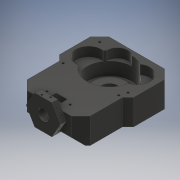
# Autodesk Inventor part: AC01
Saved by Autodesk Inventor 2017 (Build 210142000, 142)
## iProperties
Created: 2019-08-28
Part Number: AC01
Material: ABS Plastic
Document SubType Name: Modeling
Designer: Dell
Density: 1.06 g/cm^3
Appearance: Smooth - Black
Mass: 650.068 g
Surface Area: 1285.03 cm^2
Volume: 613.271 cm^3
Author: Dell
Autodesk Inventor part; units mm, degrees
ref_plane "YZ Plane" through (0, 0, 0) normal (1, 0, 0) x (0, 1, 0)
ref_plane "XZ Plane" through (0, 0, 0) normal (0, 1, 0) x (-1, 0, 0)
ref_plane "XY Plane" through (0, 0, 0) normal (0, 0, 1) x (1, 0, 0)
sketch "Sketch1" plane through (0, 0, 0) normal (0, 0, 1) x (1, 0, 0)
  circle A0 centre (0, 0) radius 17.5
  circle A1 centre (0, 0) radius 82.5
  circle A2 centre (41.5, 0) radius 2
  circle A3 centre (29.3449, 29.3449) radius 2
  circle A4 centre (0, 41.5) radius 2
  circle A5 centre (-29.3449, 29.3449) radius 2
  circle A6 centre (-41.5, 0) radius 2
  circle A7 centre (-29.3449, -29.3449) radius 2
  circle A8 centre (0, -41.5) radius 2
  circle A9 centre (29.3449, -29.3449) radius 2
  dimension "d0" = 35
  dimension "d1" = 165
  dimension "d2" = 4
  dimension "d3" = 41.5
  dimension "d6" = 360
  constraints: 10 centre point, 2 coincident, 1 horizontal alignment, 17 other
  measures "d0" diameter of A0
  measures "d1" diameter of A1
  measures "d2" diameter of A2
  measures "d3" distance of A2.centre point (0, 0)
extrude "Extrusion1" add sketch "Sketch1" along normal blind 15
sketch "Sketch5" plane through (0, 0, 15) normal (0, 0, 1) x (1, 0, 0)
  circle A0 centre (0, 0) radius 82.5 projected
  circle A1 centre (0, 0) radius 48.5
  dimension "d19" = 97
  constraints: 1 centre point
  measures "d19" diameter of A1
extrude "Extrusion4" add sketch "Sketch5" along normal blind 40
sketch "Sketch11" plane through (0, 0, 55) normal (0, 0, 1) x (1, 0, 0)
  line L0 (0, 95.2628) -> (82.5, 47.6314)
  line L1 (82.5, 47.6314) -> (82.5, -47.6314)
  line L2 (82.5, -47.6314) -> (0, -95.2628)
  line L3 (0, -95.2628) -> (-82.5, -47.6314)
  line L4 (-82.5, -47.6314) -> (-82.5, 47.6314)
  line L5 (-82.5, 47.6314) -> (0, 95.2628)
  circle A0 centre (0, 0) radius 82.5 projected
  constraints: 12 end point, 1 coincident, 1 tangent, 1 vertical alignment, 13 other
extrude "Extrusion8" add sketch "Sketch11" against normal blind 55 contours L0 A0 L5 | L0 L1 A0 | A0 L4 L5 | L1 L2 A0 | A0 L3 L4 | L2 L3 A0
sketch "Sketch16" plane through (0, 0, 15) normal (0, 0, 1) x (1, 0, 0)
  circle A0 centre (-41.5, 0) radius 2 projected
  circle A1 centre (0, 0) radius 34.5
  circle A2 centre (0, 0) radius 48.5
  line L0 (-48.5, 0) -> (-34.5, 0)
  circle A3 centre (0, 0) radius 48.5 projected
  constraints: 3 coincident, 3 horizontal alignment, 2 end point, 1 horizontal, 1 midpoint, 5 other
extrude "Extrusion11" cut sketch "Sketch16" against normal blind 8
sketch "Sketch19" plane through (0, 0, 55) normal (0, 0, 1) x (1, 0, 0)
  circle A0 centre (0, 0) radius 48.5 projected
  line L0 (0, -95.2628) -> (-82.5, -47.6314) projected
  line L1 (82.5, -47.6314) -> (0, -95.2628) projected
  line L2 (82.5, 47.6314) -> (82.5, -47.6314) projected
  line L3 (0, 95.2628) -> (82.5, 47.6314) projected
  line L4 (-82.5, 47.6314) -> (0, 95.2628) projected
  line L5 (-82.5, -47.6314) -> (-82.5, 47.6314) projected
  line L6 (0, 86.6025) -> (75, 43.3013)
  line L7 (75, 43.3013) -> (75, -43.3013)
  line L8 (75, -43.3013) -> (0, -86.6025)
  line L9 (0, -86.6025) -> (-75, -43.3013)
  line L10 (-75, -43.3013) -> (-75, 43.3013)
  line L11 (-75, 43.3013) -> (0, 86.6025)
  dimension "d58" = 150
  constraints: 12 end point, 5 other
  measures "d58" distance between parallel lines of L7 L10
extrude "Extrusion13" cut sketch "Sketch19" against normal through all contours L0 L5 L4 L3 L2 L1
sketch "Sketch20" plane through (0, 0, 0) normal (0, 0, -1) x (-1, 0, 0)
  line L0 (-75, -43.3013) -> (-75, -130)
  line L1 (-75, -130) -> (75, -130)
  line L2 (75, -43.3013) -> (75, 43.3013) projected
  line L3 (75, -130) -> (75, -43.3013)
  line L4 (-75, -43.3013) -> (0, -86.6025) projected
  line L5 (0, -86.6025) -> (75, -43.3013) projected
  line L6 (-75, -43.3013) -> (0, -86.6025)
  line L7 (0, -86.6025) -> (75, -43.3013)
  point P0 (0, 0)
  dimension "d61" = 130
  constraints: 10 end point, 2 vertical, 1 collinear, 1 horizontal
  measures "d61" distance from line of point (0, 0) L1
extrude "Extrusion14" add sketch "Sketch20" against normal blind 55
sketch "Sketch22" plane through (0, 0, 55) normal (0, 0, 1) x (1, 0, 0)
  line L0 (75, -130) -> (75, 43.3013) construction
  line L1 (75, 43.3013) -> (0, 86.6025) construction
  line L2 (0, 86.6025) -> (-75, 43.3013) construction
  line L3 (-75, 43.3013) -> (-75, -130) construction
  line L4 (-75, -130) -> (75, -130) construction
  line L5 (68, 39.2598) -> (68, -123) construction
  line L6 (68, -123) -> (-68, -123) construction
  line L7 (-68, -123) -> (-68, 39.2598) construction
  line L8 (-68, 39.2598) -> (0, 78.5196) construction
  line L9 (0, 78.5196) -> (68, 39.2598) construction
  circle A0 centre (-68, -123) radius 2
  circle A1 centre (68, -123) radius 2
  circle A2 centre (0, 78.5196) radius 2
  circle A3 centre (-68, 39.2598) radius 2
  circle A4 centre (68, 39.2598) radius 2
  circle A5 centre (-34, -123) radius 2
  circle A6 centre (34, -123) radius 2
  circle A7 centre (0, -123) radius 2
  circle A8 centre (-68, -71.8701) radius 2
  circle A9 centre (-68, -41.8701) radius 2
  circle A10 centre (-68, 0) radius 2
  circle A11 centre (68, 0) radius 2
  circle A12 centre (68, -41.8701) radius 2
  circle A13 centre (68, -71.8701) radius 2
  circle A14 centre (-34, 58.8897) radius 2
  circle A15 centre (34, 58.8897) radius 2
  point P0 (0, 0)
  point P1 (0, 0)
  dimension "d64" = 7
  dimension "d65" = 4
  dimension "d66" = 4
  dimension "d67" = 4
  dimension "d68" = 4
  dimension "d69" = 4
  dimension "d70" = 4
  dimension "d71" = 4
  dimension "d72" = 4
  dimension "d73" = 4
  dimension "d74" = 4
  dimension "d75" = 4
  dimension "d76" = 4
  dimension "d77" = 4
  dimension "d78" = 4
  dimension "d79" = 4
  dimension "d80" = 4
  dimension "d81" = 30
  constraints: 20 end point, 16 centre point, 11 coincident, 6 point on line, 5 midpoint, 3 horizontal alignment, 2 vertical alignment, 4 other
  measures "d64" distance between parallel lines of L0 L5
  measures "d65" diameter of A0
  measures "d66" diameter of A1
  measures "d67" diameter of A2
  measures "d68" diameter of A3
  measures "d69" diameter of A4
  measures "d70" diameter of A5
  measures "d71" diameter of A6
  measures "d72" diameter of A7
  measures "d73" diameter of A8
  measures "d74" diameter of A9
  measures "d75" diameter of A10
  measures "d76" diameter of A11
  measures "d77" diameter of A12
  measures "d78" diameter of A13
  measures "d79" diameter of A14
  measures "d80" diameter of A15
  measures "d81" distance of A9.centre A8.centre
extrude "Extrusion15" cut sketch "Sketch22" against normal through all contours A0 | A1 | A3 | A4 | A9 | A12 | A14 | A15
sketch "Sketch23" plane through (-75, -130, 0) normal (0, -1, 0) x (1, 0, 0)
  line L0 (28.812, 40) -> (51.906, 80)
  line L1 (51.906, 80) -> (98.094, 80)
  line L2 (98.094, 80) -> (121.188, 40)
  line L3 (121.188, 40) -> (98.094, 0)
  line L4 (98.094, 0) -> (51.906, 0)
  line L5 (51.906, 0) -> (28.812, 40)
  line L6 (150, 0) -> (0, 0) projected
  point P0 (75, 0)
  point P1 (75, 40)
  point P2 (75, 0)
  point P3 (75, 0)
  dimension "d87" = 80
  constraints: 12 end point, 3 midpoint, 1 horizontal, 1 vertical alignment, 13 other
  measures "d87" distance between parallel lines of L1 L4
extrude "Extrusion16" add sketch "Sketch23" along normal blind 13
sketch "Sketch24" plane through (-75, -143, 0) normal (0, -1, 0) x (1, 0, 0)
  line L0 (51.906, 80) -> (28.812, 40) projected
  line L1 (28.812, 40) -> (51.906, 0) projected
  line L2 (51.906, 0) -> (98.094, 0) projected
  line L3 (98.094, 0) -> (121.188, 40) projected
  line L4 (121.188, 40) -> (98.094, 80) projected
  line L5 (98.094, 80) -> (51.906, 80) projected
  line L6 (56.5248, 8) -> (38.0496, 40)
  line L7 (38.0496, 40) -> (56.5248, 72)
  line L8 (56.5248, 72) -> (93.4752, 72)
  line L9 (93.4752, 72) -> (111.9504, 40)
  line L10 (111.9504, 40) -> (93.4752, 8)
  line L11 (93.4752, 8) -> (56.5248, 8)
  point P0 (75, 0)
  dimension "d88" = 8
  constraints: 12 end point, 5 other
  measures "d88" distance between parallel lines of L1 L6
extrude "Extrusion17" cut sketch "Sketch24" against normal up to surface (13 mm away) from surface at 0
sketch "Sketch25" plane through (-75, -143, 0) normal (0, -1, 0) x (1, 0, 0)
  line L0 (111.9504, 40) -> (93.4752, 72) projected
  line L1 (93.4752, 72) -> (56.5248, 72) projected
  line L2 (56.5248, 72) -> (38.0496, 40) projected
  line L3 (38.0496, 40) -> (56.5248, 8) projected
  line L4 (56.5248, 8) -> (93.4752, 8) projected
  line L5 (93.4752, 8) -> (111.9504, 40) projected
  circle A0 centre (75, 40) radius 12
  point P0 (75, 0)
  point P1 (75, 72)
  dimension "d91" = 24
  constraints: 1 centre point, 1 horizontal alignment, 1 midpoint, 1 vertical alignment
  measures "d91" diameter of A0
extrude "Extrusion18" cut sketch "Sketch25" against normal blind 40 contours A0
sketch "Sketch26" plane through (0, 0, 55) normal (0, 0, 1) x (1, 0, 0)
  line L0 (12, -103) -> (-12, -103) projected
  line L1 (12, -143) -> (-12, -143) projected
  line L2 (12, -103) -> (-12, -103) projected
  line L3 (-12, -103) -> (12, -103)
  line L4 (12, -103) -> (12, -116)
  line L5 (12, -116) -> (-12, -116)
  line L6 (-12, -116) -> (-12, -103)
  point P0 (0, 0)
  dimension "d94" = 13
  constraints: 8 end point, 2 parallel, 1 horizontal, 1 perpendicular
  measures "d94" distance between parallel lines of L0 L5
extrude "Extrusion19" cut sketch "Sketch26" against normal blind 15
sketch "Sketch27" plane through (-36.9504, -143, 40) normal (-0.8660254, 0, 0.5) x (0.5, 0, 0.8660254)
  line L0 (17.3205, 13) -> (36.9504, 13) projected
  line L1 (17.3205, 13) -> (0, 13) projected
  line L2 (0, 0) -> (0, 13) projected
  line L3 (36.9504, 0) -> (0, 0) projected
  line L4 (36.9504, 0) -> (36.9504, 13) projected
  circle A0 centre (11.4041, 4) radius 2
  circle A1 centre (25.5463, 9) radius 2
  line L5 (11.4041, 4) -> (25.5463, 9) construction
  line L6 (0, 13) -> (36.9504, 13) projected
  point P0 (-16.1658, 143)
  point P1 (18.4752, 6.5)
  point P2 (18.4752, 13)
  point P3 (0, 6.5)
  dimension "d97" = 4
  dimension "d98" = 4
  dimension "d99" = 15
  dimension "d112" = 5
  constraints: 3 midpoint, 2 centre point, 2 end point, 1 horizontal alignment, 1 vertical alignment
  measures "d97" diameter of A0
  measures "d98" diameter of A1
  measures "d99" distance of L5.start L5.end
  measures "d112" vertical distance of L5.end L5.start
extrude "Extrusion20" cut sketch "Sketch27" against normal blind 20 contours A0 | A1
pattern_circular "Circular Pattern1" count 6 over 360 about axis through (0, -143, 40) along (0, 1, 0) of "Extrusion20"
sketch "Sketch28" plane through (0, 0, 55) normal (0, 0, 1) x (1, 0, 0)
  circle A0 centre (0, 71.6025) radius 2
  circle A1 centre (-50, -105) radius 2
  line L0 (-75, 43.3013) -> (-75, -130) projected
  line L1 (-75, -130) -> (-28.2902, -130) projected
  point P0 (0, 0)
  point P1 (0, 86.6025)
  dimension "d105" = 4
  dimension "d106" = 15
  dimension "d107" = 4
  dimension "d108" = 25
  dimension "d109" = 25
  constraints: 2 centre point, 1 vertical alignment
  measures "d105" diameter of A0
  measures "d106" distance of A0.centre point (0, 86.603)
  measures "d107" diameter of A1
  measures "d108" distance from line of L0 A1.centre
  measures "d109" distance from line of L1 A1.centre
extrude "Extrusion21" cut sketch "Sketch28" against normal through all
sketch "Sketch30" plane through (0, 0, 55) normal (0, 0, 1) x (1, 0, 0)
  circle A0 centre (0, 0) radius 48.5 construction
  line L0 (12, -103) -> (12, -116) construction
  line L1 (12, -103) -> (-12, -103) construction
  line L2 (-12, -103) -> (-12, -116) construction
  line L3 (-12, -116) -> (12, -116) construction
  line L4 (12, -143) -> (-12, -143) construction
  circle A1 centre (-50, -105) radius 2 construction
  line L5 (-17, -98) -> (17, -98) construction
  line L6 (17, -98) -> (17, -121) construction
  line L7 (17, -121) -> (-17, -121) construction
  line L8 (-17, -121) -> (-17, -98) construction
  circle A2 centre (-50, -105) radius 7 construction
  circle A3 centre (0, 0) radius 53.5 construction
  circle A4 centre (0, 71.6025) radius 2 construction
  circle A5 centre (-50, -105) radius 2 construction
  line L9 (-12, -116) -> (-12, -103) construction
  line L10 (-12, -103) -> (12, -103) construction
  line L11 (12, -103) -> (12, -116) construction
  line L12 (12, -116) -> (-12, -116) construction
  circle A6 centre (34, 58.8897) radius 2 construction
  circle A7 centre (-68, 39.2598) radius 2 construction
  circle A8 centre (-68, -123) radius 2 construction
  circle A9 centre (68, -41.8701) radius 2 construction
  circle A10 centre (68, -123) radius 2 construction
  circle A11 centre (-68, -41.8701) radius 2 construction
  circle A12 centre (-34, 58.8897) radius 2 construction
  circle A13 centre (68, 39.2598) radius 2 construction
  line L13 (0, 86.6025) -> (-75, 43.3013) construction
  line L14 (-75, 43.3013) -> (-75, -130) construction
  line L15 (-75, -130) -> (-28.2902, -130) construction
  line L16 (-28.2902, -130) -> (28.2902, -130) construction
  line L17 (28.2902, -130) -> (75, -130) construction
  line L18 (75, -130) -> (75, 43.3013) construction
  line L19 (75, 43.3013) -> (0, 86.6025) construction
  circle A14 centre (0, 0) radius 48.5 construction
  line L20 (-62, -117) -> (-62, 35.7957) construction
  line L21 (-62, 35.7957) -> (0, 71.5914) construction
  line L22 (0, 71.5914) -> (62, 35.7957) construction
  line L23 (62, 35.7957) -> (62, -117) construction
  line L24 (62, -117) -> (28.2902, -117) construction
  line L25 (28.2902, -117) -> (-28.2902, -117) construction
  line L26 (-28.2902, -117) -> (-62, -117) construction
  line L27 (-31, -58.4295) -> (-16, -67.0897)
  line L28 (-16, -67.0897) -> (-16, -84.4103)
  line L29 (-16, -84.4103) -> (-31, -93.0705)
  line L30 (-31, -93.0705) -> (-46, -84.4103)
  line L31 (-46, -84.4103) -> (-46, -67.0897)
  line L32 (-46, -67.0897) -> (-31, -58.4295)
  line L33 (31, -58.4295) -> (46, -67.0897)
  line L34 (46, -67.0897) -> (46, -84.4103)
  line L35 (46, -84.4103) -> (31, -93.0705)
  line L36 (31, -93.0705) -> (16, -84.4103)
  line L37 (16, -84.4103) -> (16, -67.0897)
  line L38 (16, -67.0897) -> (31, -58.4295)
  line L39 (0, -98) -> (-62, -98) construction
  line L40 (0, -98) -> (62, -98) construction
  line L41 (0, -53.5) -> (0, -98) construction
  point P0 (-31, -75.75)
  point P1 (31, -75.75)
  point P2 (-31, -98)
  point P3 (31, -98)
  point P4 (0, -75.75)
  dimension "d121" = 5
  dimension "d122" = 5
  dimension "d123" = 5
  dimension "d124" = 13
  dimension "d125" = 30
  constraints: 52 end point, 5 vertical alignment, 4 midpoint, 3 horizontal alignment, 3 point on line, 2 vertical, 1 centre point, 1 perpendicular, 37 other
  measures "d121" distance between parallel lines of L1 L5
  measures "d122" radial gap between concentric circles of A1 A2
  measures "d124" distance between parallel lines of L14 L20
  measures "d125" distance between parallel lines of L34 L37
extrude "Extrusion23" [suppressed]
sketch "Sketch31" plane through (0, 0, 5) normal (0, 0, 1) x (1, 0, 0)
  line L0 (-52.3536, -52.747) -> (-52.3536, -97.747)
  line L1 (-52.3536, -97.747) -> (-41.747, -108.3536)
  line L2 (-41.747, -108.3536) -> (-26.747, -108.3536)
  circle A0 centre (-52, -108) radius 2 projected
  line L3 (-52, -108) -> (-47.0503, -103.0503)
  line L4 (-26.747, -98.3536) -> (-37.6048, -98.3536)
  line L5 (-37.6048, -98.3536) -> (-42.3536, -93.6048)
  line L6 (-42.3536, -93.6048) -> (-42.3536, -52.747)
  line L7 (-52.3536, -52.747) -> (-42.3536, -52.747)
  line L8 (-26.747, -98.3536) -> (-26.747, -108.3536)
  point P0 (0, 0)
  dimension "d128" = 45
  dimension "d129" = 15
  dimension "d130" = 15
  dimension "d131" = 135
  dimension "d132" = 7
  dimension "d133" = 10
  constraints: 18 end point, 4 perpendicular, 1 horizontal, 1 midpoint, 1 vertical, 2 other
  measures "d128" distance of L0.start L0.end
  measures "d129" distance of L1.end L2.end
  measures "d130" distance of L0.end L1.end
  measures "d131" angle of L0 L1
  measures "d132" distance of L3.start L3.end
  measures "d133" distance between parallel lines of L1 L5
extrude "Extrusion24" [suppressed]
mirror "Mirror1" [suppressed]
sketch "Sketch32" plane through (0, 0, 0) normal (0, 0, -1) x (-1, 0, 0)
  circle A0 centre (0, 0) radius 33
  dimension "d139" = 66
  constraints: 1 centre point, 1 coincident
  measures "d139" diameter of A0
extrude "Extrusion25" cut sketch "Sketch32" against normal blind 2
sketch "Sketch34" plane through (0, 0, 55) normal (0, 0, 1) x (1, 0, 0)
  circle A0 centre (44.8288, 3.922) radius 27.5
  line L0 (0, 0) -> (44.8288, 3.922) construction
  line L1 (0, 0) -> (28.2722, 0) construction
  circle A1 centre (-45, 0) radius 27.5
  circle A2 centre (-14.7916, 31.7208) radius 22.5
  line L2 (-14.7916, 31.7208) -> (0, 0) construction
  dimension "d146" = 5
  dimension "d147" = 45
  dimension "d148" = 55
  dimension "d154" = 55
  dimension "d155" = 45
  dimension "d156" = 115
  dimension "d157" = 45
  dimension "d158" = 35
  constraints: 6 end point, 3 centre point, 1 horizontal, 1 horizontal alignment
  measures "d146" angle of L1 L0
  measures "d147" distance of L0.start L0.end
  measures "d148" diameter of A0
  measures "d154" diameter of A1
  measures "d155" distance of A1.centre L0.start
  measures "d156" angle of L1 L2
  measures "d157" diameter of A2
  measures "d158" distance of L2.start L0.start
extrude "Extrusion27" cut sketch "Sketch34" against normal blind 20
chamfer "Chamfer3" distance 15 angle 45 1 edges at (0, -130, 0)
sketch "Sketch35" plane through (0, 0, 55) normal (0, 0, 1) x (1, 0, 0)
  circle A0 centre (0, 71.6025) radius 2 projected
  line L0 (0, 86.6025) -> (-75, 43.3013) projected
  line L1 (-47.809, 59) -> (47.809, 59)
  line L2 (0, 86.6025) -> (75, 43.3013) projected
  line L3 (75, 43.3013) -> (0, 86.6025) projected
  line L4 (-47.809, 59) -> (0, 86.6025)
  line L5 (0, 86.6025) -> (47.809, 59)
  point P0 (0, 0)
  point P1 (0, 59)
  dimension "d159" = 27.6025
  constraints: 6 end point, 3 point on line, 1 collinear, 1 horizontal, 1 midpoint, 1 vertical alignment
  measures "d159" distance from line of L0.start L1
extrude "Extrusion28" cut sketch "Sketch35" against normal through all
sketch "Sketch36" plane through (0, 0, 55) normal (0, 0, 1) x (1, 0, 0)
  line L0 (-68.1273, 0) -> (-34.0637, 59)
  line L1 (-34.0637, 59) -> (34.0637, 59)
  line L2 (34.0637, 59) -> (68.1273, 0)
  line L3 (68.1273, 0) -> (34.0637, -59)
  line L4 (34.0637, -59) -> (-34.0637, -59)
  line L5 (-34.0637, -59) -> (-68.1273, 0)
  line L6 (32.003, 59) -> (-32.003, 59) projected
  line L7 (-34.0637, 59) -> (-68.1273, 0)
  line L8 (-68.1273, 0) -> (-34.0637, -59)
  line L9 (-34.0637, -59) -> (-75, -59)
  line L10 (-75, -115) -> (-75, 43.3013) projected
  line L11 (-75, -59) -> (-75, 43.3013)
  line L12 (-47.809, 59) -> (-75, 43.3013) projected
  line L13 (-75, 43.3013) -> (-47.809, 59)
  line L14 (-47.809, 59) -> (-34.0637, 59)
  line L15 (34.0637, -59) -> (75, -59)
  line L16 (75, 43.3013) -> (75, -115) projected
  line L17 (75, 43.3013) -> (75, -59)
  arc A0 (32.003, 59) -> (35.997, 59) centre (34, 58.8897) ccw projected
  line L18 (35.997, 59) -> (47.809, 59) projected
  line L19 (47.809, 59) -> (47.809, 59)
  line L20 (75, 43.3013) -> (47.809, 59) projected
  line L21 (75, 43.3013) -> (47.809, 59)
  line L22 (34.0637, 59) -> (47.809, 59)
  point P0 (0, 0)
  point P1 (0, 0)
  constraints: 34 end point, 7 collinear, 3 point on line, 2 horizontal, 1 coincident, 13 other
extrude "Extrusion29" cut sketch "Sketch36" along normal through all both and the other way through all contours L5 L9 L10 L12 L14 L0 | L3 L2 A0 L18 L20 L16 L15 | L22 A0 L2
sketch "Sketch37" plane through (0, 0, 55) normal (0, 0, 1) x (1, 0, 0)
  line L0 (-35.094, 57.2154) -> (-52.9235, 26.3338) projected
  line L1 (32.003, 59) -> (-32.003, 59) projected
  line L2 (50.3037, 30.8715) -> (35.094, 57.2154) projected
  arc A0 (-35.094, 57.2154) -> (-32.003, 59) centre (-34, 58.8897) ccw projected
  line L3 (-32.003, 59) -> (-34.0637, 59)
  line L4 (-34.0637, 59) -> (-35.094, 57.2154)
  line L5 (32.003, 59) -> (34.0637, 59)
  line L6 (35.094, 57.2154) -> (68.1273, 0) projected
  line L7 (34.0637, 59) -> (35.094, 57.2154)
  arc A1 (32.003, 59) -> (35.094, 57.2154) centre (34, 58.8897) ccw projected
  point P0 (0, 0)
  constraints: 8 end point, 4 collinear
extrude "Extrusion30" add sketch "Sketch37" against normal up to surface (55 mm away) from surface at 0
sketch "Sketch39" plane through (0, 0, 55) normal (0, 0, 1) x (1, 0, 0)
  line L0 (-34.0637, -59) -> (-68.1273, 0) projected
  line L1 (-68.1273, 0) -> (-75, 0)
  line L2 (-75, 0) -> (-75, -130)
  line L3 (-75, -130) -> (-68.1273, -130)
  line L4 (-68.1273, -130) -> (-68.1273, 0)
  line L5 (68.1273, 0) -> (50.3037, 30.8715) projected
  line L6 (28.2902, -130) -> (75, -130) projected
  line L7 (68.1273, 0) -> (75, 0)
  line L8 (75, 0) -> (75, -130)
  line L9 (75, -130) -> (68.1273, -130)
  line L10 (68.1273, -130) -> (68.1273, 0)
  point P0 (0, 0)
  constraints: 16 end point, 4 parallel, 2 horizontal, 2 perpendicular
extrude "Extrusion31" cut sketch "Sketch39" along normal through all both and the other way through all
sketch "Sketch40" plane through (0, 0, 55) normal (0, 0, 1) x (1, 0, 0)
  line L0 (-68.1273, 0) -> (-68.1273, -59)
  line L1 (68.1273, 0) -> (50.3037, 30.8715) projected
  line L2 (34.0637, -59) -> (68.1273, -59) projected
  line L3 (68.1273, 0) -> (68.1273, -59)
  line L4 (68.1273, -59) -> (34.0637, -59)
  line L5 (34.0637, -59) -> (68.1273, 0)
  line L6 (-34.0637, -59) -> (-68.1273, -59) projected
  line L7 (-52.9235, -26.3338) -> (-34.0637, -59) projected
  line L8 (-68.1273, 0) -> (-52.9235, -26.3338) projected
  line L9 (-68.1273, 0) -> (-34.0637, -59)
  line L10 (-68.1273, -59) -> (-34.0637, -59) projected
  line L11 (-34.0637, -59) -> (-68.1273, -59)
  point P0 (0, 0)
  constraints: 12 end point, 2 collinear, 2 vertical
extrude "Extrusion32" add sketch "Sketch40" against normal up to surface (55 mm away) from surface at 0
sketch "Sketch41" plane through (0, 0, 35) normal (0, 0, 1) x (1, 0, 0)
  arc A0 (-40.2333, 27.0837) -> (-52.9235, 26.3338) centre (-45, 0) ccw projected
  arc A1 (50.3037, 30.8715) -> (37.7197, 30.4872) centre (44.8288, 3.922) ccw projected
  arc A2 (-40.2333, 27.0837) -> (-52.9235, 26.3338) centre (-45, 0) ccw projected
  circle A3 centre (-45, 0) radius 27.5
  circle A4 centre (44.8288, 3.922) radius 27.5
  point P0 (0, 0)
  constraints: 2 coincident, 6 other
extrude "Extrusion33" cut sketch "Sketch41" along normal blind 20
sketch "Sketch42" plane through (0, 0, 55) normal (0, 0, 1) x (1, 0, 0)
  arc A0 (-40.2333, 27.0837) -> (-52.9235, 26.3338) centre (-45, 0) ccw projected
  arc A1 (50.3037, 30.8715) -> (37.7197, 30.4872) centre (44.8288, 3.922) ccw projected
  circle A2 centre (-45, 0) radius 27.5
  circle A3 centre (44.8288, 3.922) radius 27.5
  line L0 (-68.1273, 0) -> (-34.0637, 59) projected
  line L1 (-34.0637, 59) -> (-80.1273, 59)
  line L2 (-80.1273, 59) -> (-80.1273, -40)
  line L3 (-80.1273, -40) -> (-68.1273, -40)
  line L4 (-68.1273, -115) -> (-68.1273, 0) projected
  arc A4 (-52.9235, 26.3338) -> (-68.1273, -14.8787) centre (-45, 0) ccw
  line L5 (-52.9235, 26.3338) -> (-34.0637, 59)
  line L6 (-68.1273, -40) -> (-68.1273, -14.8787)
  line L7 (-34.0637, 59) -> (34.0637, 59) projected
  line L8 (-80.1273, 59) -> (-34.0637, 59)
  line L9 (-34.0637, 59) -> (-34.0637, 59)
  line L10 (34.0637, 59) -> (50.3037, 30.8715) projected
  line L11 (68.1273, 0) -> (50.3037, 30.8715) projected
  line L12 (68.1273, 0) -> (68.1273, -10.6871) projected
  line L13 (68.1273, -10.6871) -> (68.1273, -121.0041) projected
  line L14 (68.1273, -10.6871) -> (68.1273, -40)
  line L15 (68.1273, 0) -> (68.1273, -115) projected
  line L16 (68.1273, -40) -> (80.1273, -40)
  line L17 (80.1273, -40) -> (80.1273, 59)
  line L18 (42.1837, 44.9358) -> (50.3037, 30.8715)
  line L19 (34.0637, 59) -> (68.1273, 0) projected
  line L20 (80.1273, 59) -> (34.0637, 59)
  line L21 (34.0637, 59) -> (50.3037, 30.8715)
  line L22 (-34.0637, 59) -> (34.0637, 59) projected
  line L23 (34.0637, 59) -> (80.1273, 59)
  line L24 (34.0637, 59) -> (34.0637, 59)
  arc A5 (42.4407, -23.4741) -> (68.1273, -10.6871) centre (44.8288, 3.922) ccw projected
  arc A6 (42.4407, -23.4741) -> (50.3037, 30.8715) centre (44.8288, 3.922) ccw
  point P0 (0, 0)
  dimension "d172" = 40
  dimension "d177" = 12
  dimension "d178" = 12
  constraints: 30 end point, 6 point on circle, 5 collinear, 5 point on line, 3 centre point, 3 horizontal, 3 horizontal alignment, 3 perpendicular, 2 coincident, 2 concentric, 1 midpoint, 4 other
  measures "d172" distance from line of L3 A0.centre
  measures "d177" distance between parallel lines of L6 L2
  measures "d178" distance between parallel lines of L17 L14
extrude "Extrusion34" add sketch "Sketch42" against normal up to surface (55 mm away) from surface at 0 contours A2 L4 L3 L2 L1 L0 | L10 L20 L17 L16 L13 A3 | A3 L12 L11
sketch "Sketch43" plane through (0, 0, 35) normal (0, 0, 1) x (1, 0, 0)
  arc A0 (50.3037, 30.8715) -> (37.7197, 30.4872) centre (44.8288, 3.922) ccw projected
  circle A1 centre (44.8288, 3.922) radius 27.5
  point P0 (0, 0)
  constraints: 1 coincident, 3 other
extrude "Extrusion35" cut sketch "Sketch43" along normal through all
sketch "Sketch44" plane through (0, 0, 35) normal (0, 0, 1) x (1, 0, 0)
  arc A0 (-40.2333, 27.0837) -> (-40.2333, -27.0837) centre (-45, 0) ccw projected
  line L0 (-52.9235, 26.3338) -> (-68.1273, 0) projected
  line L1 (-68.1273, -14.8787) -> (-68.1273, 0) projected
  point P0 (0, 0)
extrude "Extrusion36" add sketch "Sketch44" against normal up to surface (35 mm away) from surface at 0
chamfer "Chamfer4" distance 20 angle 45 2 edges at (-80.1273, 59, 27.5) (80.1273, 59, 27.5)
chamfer "Chamfer5" distance 12 angle 45 2 edges at (-80.1273, -40, 27.5) (80.1273, -40, 27.5)
sketch "Sketch46" plane through (0, 0, 55) normal (0, 0, 1) x (1, 0, 0)
  circle A0 centre (-50, -105) radius 2 projected
  arc A1 (68.1273, -121.0041) -> (68.1273, -124.9959) centre (68, -123) ccw projected
  arc A2 (-68.1273, -124.9959) -> (-68.1273, -121.0041) centre (-68, -123) ccw projected
  line L0 (68.1273, -40) -> (68.1273, -121.0041) projected
  arc A3 (68.1273, -121.0041) -> (68.1273, -124.9959) centre (68, -123) ccw projected
  line L1 (68.1273, -121.0041) -> (68.1273, -124.9959)
  line L2 (-68.1273, -121.0041) -> (-68.1273, -40) projected
  line L3 (-68.1273, -121.0041) -> (-68.1273, -124.9959)
  point P0 (0, 0)
  constraints: 4 end point, 1 collinear, 1 vertical
extrude "Extrusion38" add sketch "Sketch46" against normal up to surface (55 mm away) from surface at 0
sketch "Sketch48" plane through (68.1273, -130, 55) normal (1, 0, 0) x (0, 0, -1)
  line L0 (40, 0) -> (47, 7) projected
  line L1 (40, 0) -> (55, 0)
  line L2 (55, 0) -> (55, 15)
  line L3 (55, 15) -> (40, 0)
  point P0 (55, 130)
  constraints: 6 end point, 1 coincident, 1 collinear, 1 horizontal, 1 perpendicular, 1 vertical alignment
extrude "Extrusion40" cut sketch "Sketch48" against normal blind 20
sketch "Sketch49" plane through (-68.1273, -130, 15) normal (-1, 0, 0) x (0, 0, 1)
  line L0 (40, 90) -> (-15, 90) projected
  line L1 (-15, 15) -> (-15, 90) projected
  line L2 (-8.9959, 8.9959) -> (-15, 15) projected
  line L3 (-15, 8.9959) -> (-8.9959, 8.9959) projected
  line L4 (-15, 5.0041) -> (-15, 8.9959) projected
  line L5 (-5.0041, 5.0041) -> (-15, 5.0041) projected
  line L6 (0, 0) -> (-5.0041, 5.0041) projected
  line L7 (40, 0) -> (0, 0) projected
  line L8 (40, 90) -> (40, 0) construction
  line L9 (-15, 90) -> (-15, 15) projected
  line L10 (-15, 15) -> (-15, 0)
  line L11 (-15, 0) -> (0, 0)
  line L12 (0, 0) -> (25, 0) projected
  line L13 (0, 0) -> (-15, 15)
  point P0 (-15, 130)
  constraints: 6 end point, 1 perpendicular, 1 point on line
extrude "Extrusion41" cut sketch "Sketch49" against normal blind 20
chamfer "Chamfer6" distance 20 angle 45 2 edges at (-68.1273, -130, 35) (68.1273, -130, 35)
sketch "Sketch50" plane through (0, 0, 35) normal (0, 0, 1) x (1, 0, 0)
  circle A0 centre (40.7839, 19.0178) radius 27.5
  line L0 (0, 0) -> (13.813, 0) construction
  line L1 (0, 0) -> (40.7839, 19.0178) construction
  dimension "d203" = 55
  dimension "d204" = 25
  dimension "d205" = 45
  constraints: 4 end point, 1 centre point, 1 horizontal
  measures "d203" diameter of A0
  measures "d204" angle of L1 L0
  measures "d205" distance of L0.start L1.end
extrude "Extrusion42" cut sketch "Sketch50" along normal through all
sketch "Sketch51" plane through (0, 0, 35) normal (0, 0, 1) x (1, 0, 0)
  arc A0 (42.4407, -23.4741) -> (25.0177, 41.5495) centre (0, 0) ccw construction
  arc A1 (42.4407, -23.4741) -> (25.0177, 41.5495) centre (0, 0) ccw projected
  arc A2 (42.4407, -23.4741) -> (68.2743, 18.2941) centre (44.8288, 3.922) ccw projected
  arc A3 (68.2743, 18.2941) -> (25.0177, 41.5495) centre (40.7839, 19.0178) ccw projected
  circle A4 centre (40.7839, 19.0178) radius 27.5 construction
  arc A5 (42.4407, -23.4741) -> (68.2743, 18.2941) centre (44.8288, 3.922) ccw
  circle A6 centre (0, 0) radius 48.5 construction
  arc A7 (47.9099, -7.5429) -> (68.2743, 18.2941) centre (40.7839, 19.0178) ccw
  arc A8 (42.4407, -23.4741) -> (47.9099, -7.5429) centre (0, 0) ccw
  constraints: 9 point on circle, 4 centre point, 2 concentric, 1 coincident
extrude "Extrusion43" add sketch "Sketch51" against normal up to surface (20 mm away) from surface at 20 contours A1 A7 A2
sketch "Sketch53" plane through (0, 0, 55) normal (0, 0, 1) x (1, 0, 0)
  line L0 (-25, -110) -> (25, -110)
  line L1 (-48.1273, -130) -> (-28.2902, -130) projected
  circle A0 centre (-25, -110) radius 2.25
  circle A1 centre (25, -110) radius 2.25
  point P0 (0, 0)
  point P1 (0, -110)
  dimension "d210" = 50
  dimension "d211" = 20
  dimension "d212" = 4.5
  dimension "d213" = 4.5
  constraints: 2 centre point, 2 coincident, 2 end point, 1 horizontal, 1 midpoint, 1 vertical alignment
  measures "d210" distance of L0.start L0.end
  measures "d211" distance between parallel lines of L1 L0
  measures "d212" diameter of A0
  measures "d213" diameter of A1
extrude "Extrusion44" cut sketch "Sketch53" against normal blind 45
sketch "Sketch54" plane through (0, 0, 55) normal (0, 0, 1) x (1, 0, 0)
  circle A0 centre (-60.1273, 39) radius 2.25
  line L0 (-60.1273, 59) -> (60.1273, 59) projected
  line L1 (-80.1273, -28) -> (-80.1273, 39) projected
  circle A1 centre (65.1273, -25) radius 2.25
  line L2 (80.1273, 39) -> (80.1273, -28) projected
  point P0 (0, 0)
  point P1 (68.1273, -40)
  dimension "d216" = 4.5
  dimension "d217" = 20
  dimension "d218" = 20
  dimension "d219" = 4.5
  dimension "d220" = 15
  dimension "d221" = 15
  constraints: 2 centre point
  measures "d216" diameter of A0
  measures "d217" distance from line of L0 A0.centre
  measures "d218" distance from line of L1 A0.centre
  measures "d219" diameter of A1
  measures "d220" distance from line of L2 A1.centre
  measures "d221" vertical distance of point (68.127, -40) A1.centre
extrude "Extrusion45" cut sketch "Sketch54" against normal blind 45
sketch "Sketch55" plane through (0, 0, 55) normal (0, 0, 1) x (1, 0, 0)
  line L0 (-60, -40) -> (60, -40) construction
  line L1 (-48.1273, -130) -> (-28.2902, -130) projected
  circle A0 centre (-60, -40) radius 2.25
  circle A1 centre (60, -40) radius 2.25
  point P0 (0, 0)
  point P1 (0, -40)
  dimension "d224" = 120
  dimension "d225" = 90
  dimension "d226" = 4.5
  dimension "d227" = 4.5
  constraints: 2 centre point, 2 coincident, 2 end point, 1 horizontal, 1 midpoint, 1 vertical alignment
  measures "d224" distance of L0.start L0.end
  measures "d225" distance between parallel lines of L1 L0
  measures "d226" diameter of A0
  measures "d227" diameter of A1
extrude "Extrusion46" cut sketch "Sketch55" against normal blind 45
body "Solid1"
